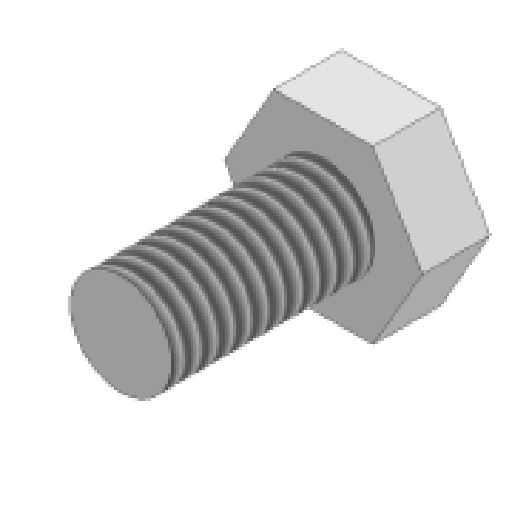
# Autodesk Inventor part: M3 screw_6mm
Saved by Autodesk Inventor 2023 (Build 270158000, 158)
## iProperties
Created: 2022-09-20
Part Number: M3 screw_6mm
Material: Generic
Document SubType Name: Modeling
Designer: CDT
Density: 1 g/cm^3
Appearance: Default
Author: CDT
Autodesk Inventor part; units mm, degrees
ref_plane "YZ Plane" through (0, 0, 0) normal (1, 0, 0) x (0, 1, 0)
ref_plane "XZ Plane" through (0, 0, 0) normal (0, 1, 0) x (-1, 0, 0)
ref_plane "XY Plane" through (0, 0, 0) normal (0, 0, 1) x (1, 0, 0)
sketch "Sketch1" plane through (0, 0, 0) normal (0, 0, 1) x (1, 0, 0)
  line L0 (1.4665, -2.54) -> (-1.4665, -2.54)
  line L1 (-1.4665, -2.54) -> (-2.9329, 0)
  line L2 (-2.9329, 0) -> (-1.4665, 2.54)
  line L3 (-1.4665, 2.54) -> (1.4665, 2.54)
  line L4 (1.4665, 2.54) -> (2.9329, 0)
  line L5 (2.9329, 0) -> (1.4665, -2.54)
  point P0 (0, 0)
  point P1 (0, 0)
  point P2 (0, -2.54)
  dimension "d1" = 2.54
  dimension "d2" = 2.54
  constraints: 12 end point, 1 coincident, 1 midpoint, 13 other
  measures "d1" distance from line of L0 point (0, 0)
  measures "d2" vertical distance of L0.end point (0, 0)
extrude "Extrusion1" add sketch "Sketch1" along normal blind 2
sketch "Sketch2" plane through (0, 0, 2) normal (0, 0, 1) x (1, 0, 0)
  circle A0 centre (0, 0) radius 1.5
  dimension "d5" = 3
  constraints: 1 centre point, 1 coincident
  measures "d5" diameter of A0
extrude "Extrusion2" add sketch "Sketch2" along normal blind 6
thread "Thread1" size "M3x0.5" class "6g" standard "ANSI Metric M Profile" full length
body "Solid1"
